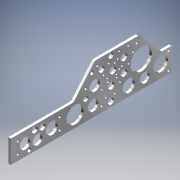
# Autodesk Inventor part: Cheese
Saved by Autodesk Inventor 2019.4 (Build 234330000, 330)
## iProperties
Created: 2019-12-06
Part Number: Cheese
Material: Aluminum 6061
Document SubType Name: Modeling
Designer: Mark
Density: 2.7 g/cm^3
Appearance: Aluminum - Flat
Mass: 518.233 g
Surface Area: 784.03 cm^2
Volume: 191.938 cm^3
Author: Mark
Autodesk Inventor part; units mm, degrees
ref_plane "YZ Plane" through (0, 0, 0) normal (1, 0, 0) x (0, 1, 0)
ref_plane "XZ Plane" through (0, 0, 0) normal (0, 1, 0) x (-1, 0, 0)
ref_plane "XY Plane" through (0, 0, 0) normal (0, 0, 1) x (1, 0, 0)
sketch "Sketch1" plane through (0, 0, 0) normal (1, 0, 0) x (0, 1, 0)
  circle A0 centre (0, 0) radius 31.75 construction
  circle A1 centre (38.1, 0) radius 6.35
  circle A2 centre (0, 0) radius 18.75 construction
  circle A3 centre (-40.8673, -58.3646) radius 52.5 construction
  circle A4 centre (-40.8673, -58.3646) radius 75 construction
  line L0 (0, 0) -> (0, -31.75) construction
  line L1 (0, 0) -> (38.1, 0) construction
  line L2 (0, 0) -> (-40.8673, -58.3646) construction
  circle A5 centre (38.1, 0) radius 30 construction
  circle A6 centre (-40.8673, -58.3646) radius 14
  circle A7 centre (-13.031, 35.8023) radius 6.35
  line L3 (0, 0) -> (-13.031, 35.8023) construction
  circle A8 centre (-13.031, 35.8023) radius 30 construction
  circle A9 centre (21.8533, 31.2097) radius 6.35
  line L4 (21.8533, 31.2097) -> (0, 0) construction
  circle A10 centre (21.8533, 31.2097) radius 30 construction
  circle A11 centre (-40.8673, 241.6354) radius 75 construction
  line L5 (-40.8673, 241.6354) -> (-40.8673, -58.3646) construction
  circle A12 centre (-40.8673, 241.6354) radius 14
  circle A13 centre (0, 0) radius 9.5
  line L6 (-64.8673, 316.6354) -> (70.1327, 316.6354)
  line L7 (70.1327, 316.6354) -> (70.1327, -133.3646)
  line L8 (70.1327, -133.3646) -> (-64.8673, -133.3646)
  line L9 (-64.8673, -133.3646) -> (-64.8673, 316.6354)
  circle A14 centre (38.1, 0) radius 25.4 construction
  circle A15 centre (38.1, 0) radius 9.7
  circle A16 centre (21.8533, 31.2097) radius 9.7
  circle A17 centre (-13.031, 35.8023) radius 9.7
  dimension "d0" = 63.5
  dimension "d1" = 12.7
  dimension "d2" = 37.5
  dimension "d3" = 105
  dimension "d4" = 150
  dimension "d5" = 90
  dimension "d6" = 35
  dimension "d7" = 60
  dimension "d8" = 28
  dimension "d9" = 12.7
  dimension "d10" = 60
  dimension "d11" = 200
  dimension "d13" = 12.7
  dimension "d14" = 145
  dimension "d15" = 60
  dimension "d16" = 150
  dimension "d17" = 300
  dimension "d18" = 28
  dimension "d19" = 19
  dimension "d20" = 135
  dimension "d21" = 450
  dimension "d22" = 24
  dimension "d23" = 75
  dimension "d24" = 50.8
  dimension "d25" = 19.4
  dimension "d26" = 19.4
  dimension "d27" = 19.4
  constraints: 20 end point, 17 centre point, 13 coincident, 3 parallel, 1 horizontal, 1 perpendicular, 1 tangent, 1 vertical, 1 vertical alignment, 5 other
  measures "d1" diameter of A1
  measures "d2" diameter of A2
  measures "d3" diameter of A3
  measures "d4" diameter of A4
  measures "d5" angle of L1 L0
  measures "d6" angle of L0 L2
  measures "d7" diameter of A5
  measures "d8" diameter of A6
  measures "d9" diameter of A7
  measures "d10" diameter of A8
  measures "d13" diameter of A9
  measures "d14" angle of L0 L4
  measures "d15" diameter of A10
  measures "d16" diameter of A11
  measures "d17" distance of L2.end L5.start
  measures "d18" diameter of A12
  measures "d19" diameter of A13
  measures "d20" distance of L7.end L8.end
  measures "d21" distance of L6.end L7.end
  measures "d22" distance from line of L5.end L9
  measures "d23" distance from line of A3.centre L8
  measures "d24" diameter of A14
  measures "d25" diameter of A15
  measures "d26" diameter of A16
  measures "d27" diameter of A17
extrude "Extrusion1" add sketch "Sketch1" along normal blind 7 contours L6 L7 L8 L9
sketch "Cheese" plane through (7, 0, 0) normal (1, 0, 0) x (0, 0, -1)
  line L0 (-316.6354, 70.1327) -> (-81.6354, 70.1327)
  line L1 (-81.6354, 70.1327) -> (-81.6354, -0.8673)
  line L2 (-81.6354, -0.8673) -> (-316.6354, -0.8673)
  line L3 (-316.6354, -0.8673) -> (-316.6354, 70.1327)
  circle A0 centre (-241.6354, -40.8673) radius 14 projected
  line L4 (-81.6354, 70.1327) -> (-141.2115, -0.8673)
  line L5 (133.3646, 70.1327) -> (-316.6354, 70.1327) projected
  line L6 (133.3646, 70.1327) -> (43.3646, 70.1327)
  line L7 (43.3646, 70.1327) -> (43.3646, -0.8673)
  line L8 (43.3646, -0.8673) -> (133.3646, -0.8673)
  line L9 (133.3646, -0.8673) -> (133.3646, 70.1327)
  circle A1 centre (58.3646, -40.8673) radius 14 projected
  line L10 (43.3646, 70.1327) -> (102.9407, -0.8673)
  circle A2 centre (-241.6354, -40.8673) radius 24
  circle A3 centre (58.3646, -40.8673) radius 24
  line L11 (-296.7727, -10.8673) -> (-252.6928, -10.8673) construction
  line L12 (-81.6354, 70.1327) -> (-141.2115, -0.8673)
  line L13 (-316.6354, 70.1327) -> (-316.6354, -64.8673) projected
  line L14 (-316.6354, -0.8673) -> (-316.6354, 70.1327)
  line L15 (-316.6354, 70.1327) -> (-81.6354, 70.1327)
  line L16 (102.9407, -0.8673) -> (43.3646, 70.1327)
  line L17 (133.3646, 70.1327) -> (43.3646, 70.1327)
  line L18 (133.3646, 70.1327) -> (133.3646, -0.8673)
  line L19 (102.9407, -0.8673) -> (133.3646, -0.8673)
  line L20 (-141.2115, -0.8673) -> (-81.6354, 70.1327)
  line L21 (-316.6354, 70.1327) -> (-81.6354, 70.1327)
  line L22 (-316.6354, 70.1327) -> (-316.6354, -0.8673)
  line L23 (-316.6354, -0.8673) -> (-141.2115, -0.8673)
  line L24 (43.3646, 70.1327) -> (133.3646, 70.1327)
  line L25 (133.3646, -0.8673) -> (133.3646, 70.1327)
  line L26 (43.3646, 70.1327) -> (102.9407, -0.8673)
  line L27 (102.9407, -0.8673) -> (133.3646, -0.8673)
  line L28 (133.3646, -64.8673) -> (133.3646, 70.1327) projected
  point P0 (0, 0)
  dimension "d30" = 40
  dimension "d32" = 40
  dimension "d33" = 71
  dimension "d34" = 71
  dimension "d35" = 40
  dimension "d36" = 90
  dimension "d37" = 40
  dimension "d38" = 48
  dimension "d39" = 48
  dimension "d44" = 125
  constraints: 52 end point, 6 perpendicular, 5 collinear, 4 parallel, 3 horizontal, 2 centre point, 2 coincident, 1 point on line, 1 vertical
  measures "d30" distance from line of A0.centre L2
  measures "d32" angle of L1 L4
  measures "d33" distance of L0.end L1.end
  measures "d34" distance from line of L0 L4.end
  measures "d35" distance from line of A1.centre L8
  measures "d36" distance between parallel lines of L9 L7
  measures "d37" angle of L7 L10
  measures "d38" diameter of A2
  measures "d39" diameter of A3
  measures "d44" distance between parallel lines of L7 L1
extrude "Extrusion2" cut sketch "Cheese" against normal blind 7 contours L0 L4 L2 L3 | L9 L8 L10 L5
sketch "Sketch3" plane through (7, 0, 0) normal (1, 0, 0) x (0, 0, -1)
  circle A0 centre (-106.8994, 15.1327) radius 3.25
  circle A1 centre (35.9037, 54.1327) radius 3.25
  circle A2 centre (68.6285, 15.1327) radius 3.25
  circle A3 centre (-296.3854, -16.8673) radius 3.25
  circle A4 centre (-296.3854, -48.8673) radius 3.25
  circle A5 centre (-74.1745, 54.1327) radius 3.25
  line L0 (-316.6354, -0.8673) -> (-316.6354, -64.8673) projected
  line L1 (-316.6354, -64.8673) -> (133.3646, -64.8673) projected
  line L2 (-141.2115, -0.8673) -> (-316.6354, -0.8673) projected
  circle A6 centre (-237.8854, -16.8673) radius 3.25
  circle A7 centre (-237.8854, -48.8673) radius 3.25
  circle A8 centre (-179.3854, -16.8673) radius 3.25
  circle A9 centre (-179.3854, -48.8673) radius 3.25
  circle A10 centre (-120.8854, -16.8673) radius 3.25
  circle A11 centre (-120.8854, -48.8673) radius 3.25
  circle A12 centre (-62.3854, -16.8673) radius 3.25
  circle A13 centre (-62.3854, -48.8673) radius 3.25
  circle A14 centre (-3.8854, -16.8673) radius 3.25
  circle A15 centre (-3.8854, -48.8673) radius 3.25
  circle A16 centre (54.6146, -16.8673) radius 3.25
  circle A17 centre (54.6146, -48.8673) radius 3.25
  circle A18 centre (113.1146, -16.8673) radius 3.25
  circle A19 centre (113.1146, -48.8673) radius 3.25
  line L3 (43.3646, 70.1327) -> (-81.6354, 70.1327) projected
  line L4 (-81.6354, 70.1327) -> (-141.2115, -0.8673) projected
  line L5 (102.9407, -0.8673) -> (43.3646, 70.1327) projected
  line L6 (133.3646, -0.8673) -> (102.9407, -0.8673) projected
  circle A20 centre (125.3646, -56.8673) radius 3.25
  line L7 (133.3646, -64.8673) -> (133.3646, -0.8673) projected
  circle A21 centre (125.3646, -8.8673) radius 3.25
  circle A22 centre (-31.2097, 21.8533) radius 25.4 construction
  circle A23 centre (-31.2097, 21.8533) radius 9.7 projected
  circle A24 centre (0, 38.1) radius 25.4 construction
  circle A25 centre (0, 38.1) radius 9.7 projected
  circle A26 centre (-35.8023, -13.031) radius 25.4 construction
  circle A27 centre (-35.8023, -13.031) radius 9.7 projected
  circle A28 centre (12.3646, 60.2873) radius 2.75
  circle A29 centre (-13.0325, 59.9017) radius 2.75
  circle A30 centre (-25.3971, 37.7144) radius 2.75
  circle A31 centre (-12.3646, 15.9127) radius 2.75
  circle A32 centre (13.0325, 16.2983) radius 2.75
  circle A33 centre (25.3971, 38.4856) radius 2.75
  circle A34 centre (-42.6354, 44.5383) radius 2.75
  circle A35 centre (-56.5684, 23.3008) radius 2.75
  circle A36 centre (-45.1427, 0.6158) radius 2.75
  circle A37 centre (-19.784, -0.8318) radius 2.75
  circle A38 centre (-5.851, 20.4057) radius 2.75
  circle A39 centre (-17.2767, 43.0908) radius 2.75
  circle A40 centre (-25.7736, -36.3673) radius 2.75
  circle A41 centre (-10.5781, -16.014) radius 2.75
  circle A42 centre (-20.6068, 7.3223) radius 2.75
  circle A43 centre (-45.831, 10.3054) radius 2.75
  circle A44 centre (-61.0265, -10.0479) radius 2.75
  circle A45 centre (-50.9978, -33.3842) radius 2.75
  point P0 (0, 0)
  dimension "d182" = 50.8
  dimension "d183" = 50.8
  dimension "d184" = 50.8
  dimension "d47" = 6.5
  dimension "d48" = 6.5
  dimension "d49" = 6.5
  dimension "d52" = 6.5
  dimension "d53" = 6.5
  dimension "d54" = 6.5
  dimension "d55" = 20.25
  dimension "d56" = 20.25
  dimension "d57" = 16
  dimension "d58" = 16
  dimension "d61" = 58.5
  dimension "d66" = 16
  dimension "d67" = 16
  dimension "d68" = 16
  dimension "d69" = 16
  dimension "d70" = 16
  dimension "d71" = 16
  dimension "d72" = 16
  dimension "d73" = 16
  dimension "d91" = 6.5
  dimension "d92" = 8
  dimension "d93" = 8
  dimension "d179" = 6.5
  dimension "d180" = 8
  dimension "d181" = 8
  dimension "d185" = 5.5
  dimension "d188" = 360
  dimension "d190" = 31
  dimension "d191" = 5.5
  dimension "d194" = 360
  dimension "d196" = 39
  dimension "d197" = 5.5
  dimension "d200" = 360
  dimension "d202" = 28.5
  constraints: 40 centre point, 1 horizontal, 79 other
  measures "d47" diameter of A0
  measures "d48" diameter of A1
  measures "d49" diameter of A2
  measures "d52" diameter of A3
  measures "d53" diameter of A4
  measures "d54" diameter of A5
  measures "d55" distance from line of L0 A3.centre
  measures "d56" distance from line of L0 A4.centre
  measures "d57" distance from line of L1 A4.centre
  measures "d58" distance from line of L2 A3.centre
  measures "d61" distance of A3.centre A6.centre
  measures "d66" distance from line of L3 A5.centre
  measures "d67" distance from line of L4 A5.centre
  measures "d68" distance from line of L4 A0.centre
  measures "d69" distance from line of L2 A0.centre
  measures "d70" distance from line of L5 A1.centre
  measures "d71" distance from line of L3 A1.centre
  measures "d72" distance from line of L5 A2.centre
  measures "d73" distance from line of L6 A2.centre
  measures "d91" diameter of A20
  measures "d92" distance from line of L7 A20.centre
  measures "d93" distance from line of L1 A20.centre
  measures "d179" diameter of A21
  measures "d180" distance from line of L7 A21.centre
  measures "d181" distance from line of L6 A21.centre
  measures "d185" diameter of A28
  measures "d190" horizontal distance of L3.start A28.centre
  measures "d191" diameter of A34
  measures "d196" horizontal distance of L3.end A34.centre
  measures "d197" diameter of A40
  measures "d202" distance from line of L1 A40.centre
extrude "Extrusion3" cut sketch "Sketch3" against normal blind 7 contours A0 | A1 | A3 | A4 | A5 | A8 | A9 | A13 | A20 | A21 | A28 | A29 | A30 | A31 | A32 | A33 | A34 | A35 | A36 | A37 | A38 | A39 | A40 | A41 | A42 | A43 | A44 | A45
sketch "Sketch6" plane through (7, 0, 0) normal (1, 0, 0) x (0, 0, -1)
  circle A0 centre (-81.6354, 10.1327) radius 15
  line L0 (43.3646, 70.1327) -> (-81.6354, 70.1327) projected
  line L1 (133.3646, -64.8673) -> (133.3646, -0.8673) projected
  line L2 (-81.6354, 70.1327) -> (-141.2115, -0.8673) projected
  circle A1 centre (48.3646, 9.1327) radius 30
  line L3 (-316.6354, -64.8673) -> (133.3646, -64.8673) projected
  circle A2 centre (103.3646, -29.8673) radius 20
  circle A3 centre (13.3646, -37.8673) radius 17.5
  circle A4 centre (-136.6354, -32.8673) radius 24
  line L4 (-316.6354, -0.8673) -> (-316.6354, -64.8673) projected
  circle A5 centre (-86.6354, -35.8673) radius 15
  line L5 (-141.2115, -0.8673) -> (-316.6354, -0.8673) projected
  circle A6 centre (-201.6354, -32.8673) radius 17
  circle A7 centre (-276.6354, -32.8673) radius 15
  circle A8 centre (-249.6354, -12.8673) radius 8.5
  circle A9 centre (-227.6354, -16.8673) radius 8.5
  circle A10 centre (-89.0925, 44.1327) radius 5
  circle A11 centre (-264.6354, -54.8673) radius 5.5
  circle A12 centre (-106.6354, -9.8673) radius 7
  circle A13 centre (-36.6354, 60.1327) radius 7.5
  circle A14 centre (-62.6354, 40.1327) radius 8.5
  circle A15 centre (-36.6354, -49.8673) radius 9
  point P0 (0, 0)
  dimension "d123" = 30
  dimension "d124" = 60
  dimension "d125" = 215
  dimension "d129" = 60
  dimension "d130" = 85
  dimension "d131" = 74
  dimension "d132" = 40
  dimension "d133" = 30
  dimension "d134" = 35
  dimension "d136" = 35
  dimension "d137" = 120
  dimension "d138" = 27
  dimension "d144" = 48
  dimension "d145" = 32
  dimension "d146" = 180
  dimension "d147" = 30
  dimension "d148" = 230
  dimension "d149" = 35
  dimension "d156" = 34
  dimension "d157" = 32
  dimension "d158" = 115
  dimension "d159" = 30
  dimension "d160" = 40
  dimension "d161" = 32
  dimension "d162" = 17
  dimension "d163" = 17
  dimension "d164" = 67
  dimension "d165" = 12
  dimension "d166" = 89
  dimension "d167" = 16
  dimension "d168" = 10
  dimension "d169" = 11
  dimension "d170" = 26
  dimension "d171" = 11
  dimension "d172" = 52
  dimension "d173" = 10
  dimension "d176" = 14
  dimension "d177" = 210
  dimension "d178" = 55
  dimension "d203" = 15
  dimension "d204" = 10
  dimension "d205" = 45
  dimension "d206" = 17
  dimension "d207" = 19
  dimension "d208" = 30
  dimension "d209" = 18
  dimension "d210" = 170
  dimension "d211" = 15
  constraints: 16 centre point
  measures "d123" diameter of A0
  measures "d124" distance from line of L0 A0.centre
  measures "d125" distance from line of L1 A0.centre
  measures "d129" diameter of A1
  measures "d130" distance from line of L1 A1.centre
  measures "d131" distance from line of L3 A1.centre
  measures "d132" diameter of A2
  measures "d133" distance from line of L1 A2.centre
  measures "d134" distance from line of L3 A2.centre
  measures "d136" diameter of A3
  measures "d137" distance from line of L1 A3.centre
  measures "d138" distance from line of L3 A3.centre
  measures "d144" diameter of A4
  measures "d145" distance from line of L3 A4.centre
  measures "d146" distance from line of L4 A4.centre
  measures "d147" diameter of A5
  measures "d148" distance from line of L4 A5.centre
  measures "d149" distance from line of L5 A5.centre
  measures "d156" diameter of A6
  measures "d157" distance from line of L3 A6.centre
  measures "d158" distance from line of L4 A6.centre
  measures "d159" diameter of A7
  measures "d160" distance from line of L4 A7.centre
  measures "d161" distance from line of A7.centre L3
  measures "d162" diameter of A8
  measures "d163" diameter of A9
  measures "d164" distance from line of L4 A8.centre
  measures "d165" distance from line of L5 A8.centre
  measures "d166" distance from line of L4 A9.centre
  measures "d167" distance from line of L5 A9.centre
  measures "d168" diameter of A10
  measures "d169" distance from line of A10.centre L2
  measures "d170" vertical distance of L0.end A10.centre
  measures "d171" diameter of A11
  measures "d172" distance from line of L4 A11.centre
  measures "d173" distance from line of L3 A11.centre
  measures "d176" diameter of A12
  measures "d177" distance from line of L4 A12.centre
  measures "d178" distance from line of L3 A12.centre
  measures "d203" diameter of A13
  measures "d204" distance from line of L0 A13.centre
  measures "d205" horizontal distance of L0.end A13.centre
  measures "d206" diameter of A14
  measures "d207" horizontal distance of L0.end A14.centre
  measures "d208" vertical distance of L0.end A14.centre
  measures "d209" diameter of A15
  measures "d210" horizontal distance of L1.start A15.centre
  measures "d211" distance from line of L3 A15.centre
extrude "Extrusion4" cut sketch "Sketch6" against normal blind 10
fillet "Fillet2" radius 10 4 edges at (3.5, -0.8673, 141.2115) (3.5, 70.1327, 81.6354) (3.5, 70.1327, -43.3646) (3.5, -0.8673, -102.9407)
sketch "Sketch7" plane through (0, -0.8673, 316.6354) normal (0, 1, 0) x (1, 0, 0)
  circle A0 centre (3.5, 10) radius 2.1
  line L0 (0, 0) -> (0, 170.7608) projected
  line L1 (7, 0) -> (0, 0) projected
  circle A1 centre (3.5, 40) radius 2.1
  circle A2 centre (4.2231, 150) radius 2.1
  point P0 (0, 316.6354)
  dimension "d213" = 4.2
  dimension "d214" = 3.5
  dimension "d215" = 10
  dimension "d221" = 4.2
  dimension "d222" = 3.5
  dimension "d223" = 40
  dimension "d224" = 4.2
  dimension "d225" = 150
  constraints: 3 centre point
  measures "d213" diameter of A0
  measures "d214" distance from line of L0 A0.centre
  measures "d215" distance from line of L1 A0.centre
  measures "d221" diameter of A1
  measures "d222" distance from line of L0 A1.centre
  measures "d223" distance from line of L1 A1.centre
  measures "d224" diameter of A2
  measures "d225" distance from line of L1 A2.centre
extrude "Extrusion5" cut sketch "Sketch7" against normal blind 10
sketch "Sketch8" plane through (0, -64.8673, 316.6354) normal (0, 0, 1) x (1, 0, 0)
  line L0 (0, 0) -> (7, 0) projected
  line L1 (7, 64) -> (0, 64) projected
  line L2 (7, 0) -> (0, 0)
  line L3 (0, 0) -> (0, 64)
  line L4 (0, 64) -> (7, 64)
  line L5 (7, 64) -> (7, 0)
  point P0 (0, 64.8673)
  dimension "d226" = 7
  dimension "d227" = 64
  constraints: 8 end point, 2 parallel, 1 horizontal, 1 perpendicular
  measures "d226" distance of L1.end L4.end
  measures "d227" distance of L2.end L1.end
extrude "Extrusion6" add sketch "Sketch8" along normal blind 200
equation "\"d9\" = d1"
equation "\"d13\" = d1"
equation "\"d14\" = 0.5 * d5 + 0.5 * d11"
equation "\"d16\" = d4"
equation "\"d18\" = d8"
equation "\"d26\" = d25"
equation "\"d27\" = d25"
equation "\"d34\" = d33"
equation "\"d35\" = d30"
equation "\"d56\" = d55"
equation "\"d58\" = d57"
body "Solid1"
